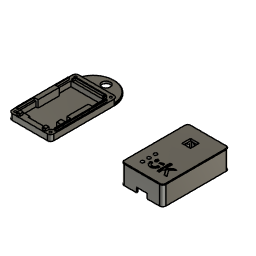
krabka_adam_v7 (Autodesk Fusion 360 design; units mm, degrees)
Autodesk Fusion 360 part; units mm, degrees
sketch "Sketch1" plane through (0, 0, 0) normal (0, 0, 1) x (1, 0, 0)
  line L0 (3.8, 1.2) -> (3.8, 2.7)
  line L1 (3.8, 2.7) -> (10.8, 2.7)
  line L2 (10.8, 2.7) -> (10.8, 1.2)
  line L3 (32.3, 10.7) -> (28, 10.7)
  line L4 (28, 10.7) -> (28, 14.9)
  line L5 (28, 14.9) -> (32.3, 14.9)
  line L6 (1.2, 50.8) -> (32.3, 50.8)
  line L7 (-0.4, 38) -> (3.2, 38)
  line L8 (3.2, 38) -> (3.2, 18)
  line L9 (3.2, 18) -> (-0.4, 18)
  line L10 (33.9, 18) -> (30.3, 18)
  line L11 (30.3, 18) -> (30.3, 38)
  line L12 (30.3, 38) -> (33.9, 38)
  line L13 (1.2, 50.8) -> (1.2, 38)
  line L14 (1.2, 18) -> (1.2, 2.5284)
  line L15 (32.3, 38) -> (32.3, 50.8)
  line L16 (32.3, 14.9) -> (32.3, 18)
  line L17 (2.7981, 1.2) -> (3.8, 1.2)
  line L18 (1.6, 53.5467) -> (1.6, 51.2)
  line L19 (1.6, 51.2) -> (2.8, 51.2)
  line L20 (2.8, 51.2) -> (2.8, 53.2)
  line L21 (2.8, 53.2) -> (30.7, 53.2)
  line L22 (30.7, 53.2) -> (30.7, 51.2)
  line L23 (30.7, 51.2) -> (31.9, 51.2)
  line L24 (31.9, 51.2) -> (31.9, 53.5467)
  line L25 (30.9, 54.4) -> (2.6, 54.4)
  circle A0 centre (33.3, -0.3) radius 2
  circle A1 centre (0.2, -0.3) radius 2
  line L26 (0.2, -3.3) -> (33.3, -3.3)
  circle A2 centre (33.3, 56.2) radius 2
  circle A3 centre (0.2, 56.2) radius 2
  line L27 (0.2, 59.2) -> (33.3, 59.2)
  line L28 (36.3, 56.2) -> (36.3, -0.3)
  line L29 (-2.8, -0.3) -> (-2.8, 56.2)
  arc A4 (32.3, 2.5284) -> (30.7019, 1.2) centre (33.3, -0.3) ccw
  arc A5 (33.3, -3.3) -> (36.3, -0.3) centre (33.3, -0.3) ccw
  line L30 (10.8, 1.2) -> (30.7019, 1.2)
  line L31 (32.3, 2.5284) -> (32.3, 10.7)
  arc A6 (2.7981, 1.2) -> (1.2, 2.5284) centre (0.2, -0.3) ccw
  arc A7 (-2.8, -0.3) -> (0.2, -3.3) centre (0.2, -0.3) ccw
  arc A8 (0.2, 59.2) -> (-2.8, 56.2) centre (0.2, 56.2) ccw
  arc A9 (1.6, 53.5467) -> (2.6, 54.4) centre (0.2, 56.2) ccw
  arc A10 (30.9, 54.4) -> (31.9, 53.5467) centre (33.3, 56.2) ccw
  arc A11 (36.3, 56.2) -> (33.3, 59.2) centre (33.3, 56.2) ccw
  line L32 (3.2, 53.2) -> (30.3, 53.2)
  line L33 (30.3, 1.2) -> (3.2, 1.2)
  circle A12 centre (33.3, 56.2) radius 1.05
  circle A13 centre (0.2, 56.2) radius 1.05
  circle A14 centre (0.2, -0.3) radius 1.05
  circle A15 centre (33.3, -0.3) radius 1.05
  circle A16 centre (16.75, 68.2) radius 4
  line L34 (16.75, 59.2) -> (16.75, 68.2) construction
  arc A17 (36.3, 56.2) -> (-2.8, 56.2) centre (16.75, 56.2) ccw
  line L35 (35.1, 50.8) -> (35.1, 2.5284)
  line L36 (-1.6, 2.5284) -> (-1.6, 50.8)
  line L37 (-0.4, 50.8) -> (-1.6, 50.8)
  line L38 (-0.4, 2.5284) -> (-1.6, 2.5284)
  line L39 (33.9, 50.8) -> (35.1, 50.8)
  line L40 (33.9, 2.5284) -> (35.1, 2.5284)
  line L41 (3.2, -0.9) -> (3.2, -2.1)
  line L42 (30.3, -0.9) -> (30.3, -2.1)
  line L43 (33.9, 50.8) -> (33.9, 38)
  line L44 (33.9, 18) -> (33.9, 2.5284)
  line L45 (-0.4, 2.5284) -> (-0.4, 18)
  line L46 (-0.4, 38) -> (-0.4, 50.8)
  line L47 (3.2, -0.9) -> (3.2, 1.2)
  line L48 (30.3, -0.9) -> (30.3, 1.2)
  line L49 (141.3, 56.2) -> (141.3, -0.3)
  line L50 (102.2, -0.3) -> (102.2, 56.2)
  arc A18 (138.3, -3.3) -> (141.3, -0.3) centre (138.3, -0.3) ccw
  line L51 (105.2, -3.3) -> (138.3, -3.3)
  arc A19 (141.3, 56.2) -> (138.3, 59.2) centre (138.3, 56.2) ccw
  line L52 (105.2, 59.2) -> (138.3, 59.2)
  arc A20 (105.2, 59.2) -> (102.2, 56.2) centre (105.2, 56.2) ccw
  arc A21 (102.2, -0.3) -> (105.2, -3.3) centre (105.2, -0.3) ccw
  circle A22 centre (138.3, -0.3) radius 0.95
  circle A23 centre (105.2, -0.3) radius 0.95
  circle A24 centre (105.2, 56.2) radius 0.95
  circle A25 centre (138.3, 56.2) radius 0.95
  line L53 (103.4, 1.5) -> (103.4, 54.4)
  line L54 (107, -2.1) -> (136.5, -2.1)
  line L55 (140.1, 54.4) -> (140.1, 1.5)
  line L56 (107, 58) -> (136.5, 58)
  line L57 (105.2, 1.5) -> (103.4, 1.5)
  line L58 (107, -0.3) -> (107, -2.1)
  arc A26 (107, -0.3) -> (105.2, 1.5) centre (105.2, -0.3) ccw
  line L59 (140.1, 1.5) -> (138.3, 1.5)
  line L60 (136.5, -0.3) -> (136.5, -2.1)
  arc A27 (138.3, 1.5) -> (136.5, -0.3) centre (138.3, -0.3) ccw
  line L61 (140.1, 54.4) -> (138.3, 54.4)
  line L62 (136.5, 56.2) -> (136.5, 58)
  arc A28 (136.5, 56.2) -> (138.3, 54.4) centre (138.3, 56.2) ccw
  line L63 (107, 58) -> (107, 56.2)
  line L64 (105.2, 54.4) -> (103.4, 54.4)
  arc A29 (105.2, 54.4) -> (107, 56.2) centre (105.2, 56.2) ccw
  circle A30 centre (112.35, 6.7) radius 1.55
  circle A31 centre (112.35, 12.8) radius 1.55
  circle A32 centre (112.35, 18.9) radius 1.55
  line L65 (116, 48) -> (124, 48)
  line L66 (124, 48) -> (124, 40)
  line L67 (124, 40) -> (116, 40)
  line L68 (116, 40) -> (116, 48)
  line L69 (6.2, 1.2) -> (6.2, -2.1)
  line L70 (27.3, 1.2) -> (27.3, -2.1)
  line L71 (3.2, -2.1) -> (6.2, -2.1)
  line L72 (27.3, -2.1) -> (30.3, -2.1)
  dimension "d9" = 2.6
  dimension "d10" = 7
  dimension "d11" = 1.5
  dimension "d12" = 9.5
  dimension "d14" = 4.2
  dimension "d16" = 2
  dimension "d18" = 20
  dimension "d19" = 20
  dimension "d20" = 16.8
  dimension "d21" = 16.8
  dimension "d28" = 1.2
  dimension "d29" = 1.2
  dimension "d32" = 1.2
  dimension "d35" = 2.4
  dimension "d37" = 0.4
  dimension "d46" = 6
  dimension "d47" = 4
  dimension "d48" = 6
  dimension "d49" = 4
  dimension "d50" = 6
  dimension "d51" = 4
  dimension "d52" = 6
  dimension "d53" = 4
  dimension "d54" = 0.3606
  dimension "d55" = 0.2
  dimension "d56" = 2.8
  dimension "d57" = 33.1
  dimension "d58" = 4
  dimension "d59" = 8.3
  dimension "d61" = 4
  dimension "d62" = 56.5
  dimension "d63" = 3
  dimension "d64" = 4.4
  dimension "d66" = 4
  dimension "d67" = 4.4
  dimension "d72" = 2.1
  dimension "d73" = 2.1
  dimension "d74" = 2.1
  dimension "d75" = 2.1
  dimension "d81" = 8
  dimension "d83" = 9
  dimension "d88" = 1.2
  dimension "d89" = 2.8284
  dimension "d90" = 5.4
  dimension "d92" = 1.2
  dimension "d93" = 2.8284
  dimension "d94" = 5.4
  dimension "d95" = 1.2
  dimension "d97" = 3
  dimension "d98" = 3
  dimension "d100" = 3.6
  dimension "d156" = 105.2
  dimension "d157" = 56.2
  dimension "d158" = 105.2
  dimension "d159" = 3
  dimension "d160" = 3
  dimension "d161" = 3
  dimension "d162" = 3
  dimension "d178" = 56.5
  dimension "d179" = 33.1
  dimension "d180" = 56.5
  dimension "d181" = 33.1
  dimension "d182" = 39.1
  dimension "d183" = 62.5
  dimension "d184" = 33.1
  dimension "d185" = 33.1
  dimension "d186" = 1.9
  dimension "d187" = 1.9
  dimension "d188" = 1.9
  dimension "d189" = 1.9
  dimension "d201" = 10.15
  dimension "d202" = 3.1
  dimension "d203" = 10
  dimension "d204" = 6.1
  dimension "d205" = 6.1
  dimension "d206" = 10.15
  dimension "d207" = 10.15
  dimension "d209" = 13.8
  dimension "d210" = 8
  dimension "d211" = 8
  dimension "d214" = 43.3
  dimension "d224" = 3
  dimension "d225" = 3
  constraint perpendicular L0 L17
  constraint perpendicular L0 L1
  constraint coincident L2.end L17
  constraint perpendicular L2 L17
  constraint perpendicular L3 L4
  constraint perpendicular L4 L5
  constraint perpendicular L7 L13
  constraint perpendicular L7 L8
  constraint coincident L14.start L13
  constraint perpendicular L9 L13
  constraint perpendicular L10 L11
  constraint collinear L13 L14
  constraint collinear L17 L30
  constraint perpendicular L6 L18
  constraint perpendicular L18 L19
  constraint perpendicular L19 L20
  constraint perpendicular L20 L21
  constraint perpendicular L21 L22
  constraint perpendicular L22 L23
  constraint perpendicular L23 L24
  constraint horizontal L25
  constraint equal L20 L22
  constraint tangent L11 A4
  constraint tangent L1 A4
  constraint concentric A0 A4
  constraint concentric A1 A6
  constraint tangent L1 A6
  constraint tangent L8 A6
  constraint horizontal L26
  constraint tangent L26 A6
  constraint coincident L26.end A4
  constraint concentric A2 A10
  constraint concentric A3 A8
  constraint tangent L11 A10
  constraint tangent L21 A10
  constraint tangent L21 A8
  constraint tangent L8 A8
  constraint vertical L29
  constraint horizontal L27
  constraint vertical L28
  constraint tangent L28 A4
  constraint tangent L27 A10
  constraint tangent L29 A8
  constraint coincident L29.start A6
  constraint coincident L28.start A10
  constraint concentric A4 A5
  constraint concentric A6 A7
  constraint concentric A8 A9
  constraint concentric A10 A11
  constraint horizontal L32
  constraint horizontal L33
  constraint coincident L30 L33.start
  constraint coincident L21 L32.start
  constraint concentric A11 A12
  constraint concentric A8 A13
  constraint concentric A7 A14
  constraint concentric A4 A15
  constraint midpoint L27 L34.start
  constraint coincident A16.centre L34.end
  constraint perpendicular L27 L34
  constraint tangent A11 A17
  constraint perpendicular L36 L37
  constraint perpendicular L36 L38
  constraint perpendicular L35 L39
  constraint perpendicular L35 L40
  constraint perpendicular L41 L71
  constraint perpendicular L42 L71
  constraint coincident L7.start L45
  constraint coincident L13.end L7
  constraint coincident L14.start L9
  constraint coincident L10.start L43
  constraint coincident L16.end L10
  constraint coincident L15.start L12
  constraint collinear L43 L44
  constraint collinear L45 L46
  constraint perpendicular L33 L47
  constraint perpendicular L30 L48
  constraint horizontal L51
  constraint horizontal L52
  constraint vertical L49
  constraint tangent L50 A20
  constraint concentric A18 A22
  constraint concentric A21 A23
  constraint concentric A20 A24
  constraint concentric A19 A25
  constraint concentric A20 A29
  constraint concentric A21 A26
  constraint concentric A18 A27
  constraint concentric A19 A28
  constraint tangent L55 A27
  constraint tangent L54 A26
  constraint tangent L56 A29
  constraint tangent L53 A29
  constraint tangent L53 A26
  constraint tangent L54 A27
  constraint tangent L55 A28
  constraint tangent L56 A28
  constraint perpendicular L53 L57
  constraint perpendicular L54 L58
  constraint tangent L58 A26
  constraint tangent L57 A26
  constraint perpendicular L55 L59
  constraint perpendicular L54 L60
  constraint tangent L59 A27
  constraint tangent L60 A27
  constraint perpendicular L55 L61
  constraint perpendicular L56 L62
  constraint tangent L62 A28
  constraint tangent L61 A28
  constraint perpendicular L56 L63
  constraint perpendicular L53 L64
  constraint tangent L64 A29
  constraint tangent L63 A29
  constraint equal A30 A31
  constraint equal A30 A32
  constraint horizontal L65
  constraint vertical L66
  constraint horizontal L67
  constraint vertical L68
  constraint coincident L33 L69.start
  constraint perpendicular L69 L71
  constraint coincident L33 L70.start
  constraint coincident L70.end L71
  constraint perpendicular L70 L71
  constraint collinear L71 L72
  measures "d9" distance of L0 L13
  measures "d10" distance of L0.end L1.end
  measures "d11" distance of L1 L17
  measures "d12" distance of L3 L17
  measures "d14" distance of L3.end L4.end
  measures "d16" distance of L8 L13
  measures "d18" distance of L7.end L8.end
  measures "d19" distance of L10.end L11.end
  measures "d20" distance of L9 L17
  measures "d21" distance of L10 L17
  measures "d28" distance of L18 L20
  measures "d29" distance of L22 L24
  measures "d32" distance of L21 L25
  measures "d35" distance of L6 L21
  measures "d37" distance of L6 L23
  measures "d46" diameter of A4
  measures "d47" diameter of A0
  measures "d48" diameter of A6
  measures "d49" diameter of A1
  measures "d50" diameter of A10
  measures "d51" diameter of A2
  measures "d52" diameter of A8
  measures "d53" diameter of A3
  measures "d54" distance of origin A1.centre
  measures "d55" horizontal distance of origin A1.centre
  measures "d56" distance of origin L29
  measures "d57" distance of A1.centre A0.centre
  measures "d58" distance of L28 L31
  measures "d59" distance of L4 L28
  measures "d61" distance of L16 L28
  measures "d62" distance of A0.centre A2.centre
  measures "d63" radius of A9
  measures "d64" distance of L24 L28
  measures "d66" distance of L15 L28
  measures "d67" distance of L18 L29
  measures "d72" diameter of A12
  measures "d73" diameter of A13
  measures "d74" diameter of A14
  measures "d75" diameter of A15
  measures "d81" diameter of A16
  measures "d83" distance of L27 A16.centre
  measures "d88" distance of L36 L45
  measures "d89" distance of A1.centre L38
  measures "d90" distance of A3.centre L37
  measures "d92" distance of L35 L43
  measures "d93" distance of A0.centre L40
  measures "d94" distance of A2.centre L39
  measures "d95" distance of L26 L71
  measures "d97" distance of A1.centre L41
  measures "d98" distance of A0.centre L42
  measures "d100" distance of L11.end L12.end
  measures "d156" horizontal distance of origin A21.centre
  measures "d157" vertical distance of origin A20.centre
  measures "d158" horizontal distance of origin A20.centre
  measures "d159" radius of A20
  measures "d160" radius of A21
  measures "d161" radius of A18
  measures "d162" radius of A19
  measures "d178" distance of A21.centre A20.centre
  measures "d179" distance of A18.centre A21.centre
  measures "d180" distance of A18.centre A19.centre
  measures "d181" distance of A20.centre A19.centre
  measures "d182" distance of L49 L50
  measures "d183" distance of L51 L52
  measures "d184" distance of L51.start A18.start
  measures "d185" distance of L52.start A19.end
  measures "d186" diameter of A22
  measures "d187" diameter of A23
  measures "d188" diameter of A24
  measures "d189" diameter of A25
  measures "d201" distance of L50 A30.centre
  measures "d202" diameter of A30
  measures "d203" distance of L51 A30.centre
  measures "d204" vertical distance of A30.centre A31.centre
  measures "d205" distance of A31.centre A32.centre
  measures "d206" distance of L50 A31.centre
  measures "d207" distance of L50 A32.centre
  measures "d209" distance of L50 L68
  measures "d210" distance of L65 L67
  measures "d211" distance of L66 L68
  measures "d214" distance of L51 L67
  measures "d224" distance of L48 L70
  measures "d225" distance of L47 L69
extrude "Extrude6" add sketch "Sketch1" along normal blind 6 contours L17 L33 L41 L47 L69 L71 | L0 L1 L2 L33 | L30 L33 L42 L48 L70 L72 | L7 L8 L9 L36 L37 L38 L45 L46 | L10 L11 L12 L35 L39 L40 L43 L44 | L18 L19 L20 L21 L22 L23 L24 L25 A9 A10 L32 | L26 L27 L28 L29 A5 A7 A8 A11 makes body 1
extrude "Extrude7" add sketch "Sketch1" along normal blind 8 contours L17 L33 L41 L47 L69 L71 | L30 L33 L42 L48 L70 L72 | L7 L8 L9 L36 L37 L38 L45 L46 | L10 L11 L12 L35 L39 L40 L43 L44 | L18 L19 L20 L21 L22 L23 L24 L25 A9 A10 L32 bodies 1
extrude "Extrude8" add sketch "Sketch1" along normal blind 3.8 from surface at 2.2 contours A0 | A1 | A2 | A3 bodies 1
extrude "Extrude9" add sketch "Sketch1" along normal blind 1.2 contours L0 L1 L2 L3 L4 L5 L6 L7 L8 L9 L10 L11 L12 L13 L14 L15 L16 L17 A4 L30 L31 A6 L33 bodies 1
extrude "Extrude10" add sketch "Sketch1" along normal blind 2 contours L27 A8 A11 A17 bodies 1
chamfer "Chamfer1" distance 0.5 angle 45 6 edges at (36.3, 27.95, 0) (35.4213, -2.4213, 0) (16.75, -3.3, 0) (-1.9213, -2.4213, 0) (-2.8, 27.95, 0) (16.75, 75.75, 0) on bodies 1
chamfer "Chamfer1" distance 0.5 angle 45 1 edges at (16.75, 75.75, 2) on bodies 1
chamfer "Chamfer2" distance 0.5 angle 45 9 edges at (35.1, 26.6642, 8) (4.7, -2.1, 8) (28.8, -2.1, 8) (-1.6, 26.6642, 8) (16.75, 54.4, 8) (31.9, 52.3734, 8) (31.3527, 53.9179, 8) (2.1473, 53.9179, 8) (1.6, 52.3734, 8) on bodies 1
extrude "Extrude11" add sketch "Sketch1" along normal blind 2 from surface at 16 separate body contours L53 L54 L55 L56 L57 L58 A26 L59 L60 A27 L61 L62 A28 L63 L64 A29 makes body 2
extrude "Extrude12" add sketch "Sketch1" along normal blind 18 contours L49 L50 A18 L51 A19 L52 A20 A21 bodies 2
extrude "Extrude13" add sketch "Sketch1" along normal blind 3 from surface at 15 contours A22 | A23 | A24 | A25 bodies 2
sketch "Sketch3" plane through (0, 0, 18) normal (0, 0, 1) x (-1, 0, 0)
  arc A0 (-105.2, -59.2) -> (-102.2, -56.2) centre (-105.2, -56.2) ccw
  line L0 (-102.2, -56.2) -> (-102.2, 0.3)
  arc A1 (-102.2, 0.3) -> (-105.2, 3.3) centre (-105.2, 0.3) ccw
  line L1 (-105.2, 3.3) -> (-138.3, 3.3)
  arc A2 (-138.3, 3.3) -> (-141.3, 0.3) centre (-138.3, 0.3) ccw
  line L2 (-141.3, 0.3) -> (-141.3, -56.2)
  arc A3 (-141.3, -56.2) -> (-138.3, -59.2) centre (-138.3, -56.2) ccw
  line L3 (-138.3, -59.2) -> (-105.2, -59.2)
  line L4 (-124, -40) -> (-116, -40)
  line L5 (-116, -40) -> (-116, -48)
  line L6 (-116, -48) -> (-124, -48)
  line L7 (-124, -48) -> (-124, -40)
  circle A4 centre (-112.35, -18.9) radius 1.55
  circle A5 centre (-112.35, -12.8) radius 1.55
  circle A6 centre (-112.35, -6.7) radius 1.55
  line L8 (-115.8427, -12.1922) -> (-115.8427, -18.4226)
  line L9 (-115.8427, -18.4226) -> (-121.233, -18.4226)
  line L10 (-121.233, -18.4226) -> (-126.6233, -18.4226)
  line L11 (-126.6233, -18.4226) -> (-126.6233, -12.2972)
  line L12 (-126.6233, -12.2972) -> (-126.6233, -6.1718)
  line L13 (-126.6233, -6.1718) -> (-127.6384, -6.1718)
  line L14 (-127.6384, -6.1718) -> (-128.6535, -6.1718)
  line L15 (-128.6535, -6.1718) -> (-128.6535, -7.7829)
  line L16 (-128.6535, -7.7829) -> (-128.6535, -9.394)
  line L17 (-128.6535, -9.394) -> (-129.2896, -10.0055)
  spline S0 degree 3 poles (-129.2896, -10.0055) (-129.6394, -10.3419) (-129.9466, -10.6238) (-129.9721, -10.6319) knots 0 0 0 0 1 1 1 1
  spline S1 degree 3 poles (-129.9721, -10.6319) (-129.9976, -10.6401) (-130.2421, -10.3408) (-130.5154, -9.9669) knots 0 0 0 0 1 1 1 1
  spline S2 degree 3 poles (-130.5154, -9.9669) (-130.7887, -9.593) (-131.5271, -8.5861) (-132.1565, -7.7294) knots 0 0 0 0 1 1 1 1
  line L18 (-132.1565, -7.7294) -> (-133.3007, -6.1718)
  line L19 (-133.3007, -6.1718) -> (-134.5123, -6.1718)
  spline S3 degree 3 poles (-134.5123, -6.1718) (-135.5426, -6.1718) (-135.7239, -6.1561) (-135.7239, -6.0668) knots 0 0 0 0 1 1 1 1
  spline S4 degree 3 poles (-135.7239, -6.0668) (-135.7239, -5.974) (-134.5727, -5.9618) (-125.7833, -5.9618) knots 0 0 0 0 1 1 1 1
  line L20 (-125.7833, -5.9618) -> (-115.8427, -5.9618)
  line L21 (-115.8427, -5.9618) -> (-115.8427, -12.1922)
  spline S5 degree 3 poles (-121.399, -6.1362) (-122.2006, -6.306) (-122.8682, -6.6822) (-123.5081, -7.3247) knots 0 0 0 0 1 1 1 1
  spline S6 degree 3 poles (-123.5081, -7.3247) (-124.3306, -8.1504) (-124.6782, -8.9335) (-124.7599, -10.1446) knots 0 0 0 0 1 1 1 1
  line L22 (-124.7599, -10.1446) -> (-124.7988, -10.7221)
  line L23 (-124.7988, -10.7221) -> (-123.7605, -10.7221)
  line L24 (-123.7605, -10.7221) -> (-122.7222, -10.7221)
  line L25 (-122.7222, -10.7221) -> (-122.6875, -10.0602)
  spline S7 degree 3 poles (-122.6875, -10.0602) (-122.6321, -9.0009) (-122.2578, -8.4125) (-121.3762, -7.999) knots 0 0 0 0 1 1 1 1
  spline S8 degree 3 poles (-121.3762, -7.999) (-121.0433, -7.8429) (-120.8931, -7.8169) (-120.3219, -7.8169) knots 0 0 0 0 1 1 1 1
  spline S9 degree 3 poles (-120.3219, -7.8169) (-119.7105, -7.8169) (-119.6174, -7.8358) (-119.1883, -8.0469) knots 0 0 0 0 1 1 1 1
  spline S10 degree 3 poles (-119.1883, -8.0469) (-118.3974, -8.4359) (-118.0175, -9.0706) (-117.9588, -10.1013) knots 0 0 0 0 1 1 1 1
  line L26 (-117.9588, -10.1013) -> (-117.924, -10.7119)
  line L27 (-117.924, -10.7119) -> (-117.4258, -10.7571)
  spline S11 degree 3 poles (-117.4258, -10.7571) (-117.1519, -10.7819) (-116.7072, -10.7921) (-116.4377, -10.7797) knots 0 0 0 0 1 1 1 1
  line L28 (-116.4377, -10.7797) -> (-115.9477, -10.7571)
  line L29 (-115.9477, -10.7571) -> (-115.9527, -10.1217)
  spline S12 degree 3 poles (-115.9527, -10.1217) (-115.9619, -8.9519) (-116.2911, -8.171) (-117.136, -7.3146) knots 0 0 0 0 1 1 1 1
  spline S13 degree 3 poles (-117.136, -7.3146) (-117.7707, -6.6712) (-118.3969, -6.3164) (-119.2079, -6.1405) knots 0 0 0 0 1 1 1 1
  spline S14 degree 3 poles (-119.2079, -6.1405) (-119.8026, -6.0116) (-120.8016, -6.0096) (-121.399, -6.1361) knots 0 0 0 0 1 1 1 1
  line L30 (-121.399, -6.1361) -> (-121.399, -6.1362)
  spline S15 degree 3 poles (-118.4353, -12.7518) (-118.7578, -12.8414) (-119.1688, -13.2675) (-119.3049, -13.6536) knots 0 0 0 0 1 1 1 1
  spline S16 degree 3 poles (-119.3049, -13.6536) (-119.5496, -14.3477) (-119.3519, -15.2268) (-118.8575, -15.6428) knots 0 0 0 0 1 1 1 1
  spline S17 degree 3 poles (-118.8575, -15.6428) (-117.7656, -16.5616) (-116.4588, -14.9288) (-117.1377, -13.4939) knots 0 0 0 0 1 1 1 1
  spline S18 degree 3 poles (-117.1377, -13.4939) (-117.3442, -13.0573) (-117.4897, -12.9124) (-117.8507, -12.7837) knots 0 0 0 0 1 1 1 1
  spline S19 degree 3 poles (-117.8507, -12.7837) (-118.1784, -12.6668) (-118.1374, -12.669) (-118.4353, -12.7518) knots 0 0 0 0 1 1 1 1
  spline S20 degree 3 poles (-122.7519, -13.2792) (-124.29, -13.4482) (-124.8198, -13.5156) (-124.8501, -13.5459) knots 0 0 0 0 1 1 1 1
  spline S21 degree 3 poles (-124.8501, -13.5459) (-124.8734, -13.5691) (-124.5803, -14.8903) (-124.4874, -15.1807) knots 0 0 0 0 1 1 1 1
  spline S22 degree 3 poles (-124.4874, -15.1807) (-124.4694, -15.2371) (-123.9446, -15.0924) (-122.8644, -14.7335) knots 0 0 0 0 1 1 1 1
  spline S23 degree 3 poles (-122.8644, -14.7335) (-121.9864, -14.4417) (-121.2547, -14.1914) (-121.2385, -14.1773) knots 0 0 0 0 1 1 1 1
  spline S24 degree 3 poles (-121.2385, -14.1773) (-121.2037, -14.1471) (-121.3637, -13.244) (-121.4199, -13.1531) knots 0 0 0 0 1 1 1 1
  spline S25 degree 3 poles (-121.4199, -13.1531) (-121.441, -13.1189) (-121.5319, -13.1094) (-121.6219, -13.132) knots 0 0 0 0 1 1 1 1
  spline S26 degree 3 poles (-121.6219, -13.132) (-121.7119, -13.1546) (-122.2204, -13.2208) (-122.7519, -13.2792) knots 0 0 0 0 1 1 1 1
  spline S27 degree 3 poles (-134.5821, -7.8023) (-133.9734, -8.6574) (-133.3848, -9.483) (-133.2742, -9.637) knots 0 0 0 0 1 1 1 1
  spline S28 degree 3 poles (-133.2742, -9.637) (-133.1635, -9.7911) (-132.7231, -10.4053) (-132.2955, -11.0021) knots 0 0 0 0 1 1 1 1
  line L31 (-132.2955, -11.0021) -> (-131.5181, -12.0872)
  line L32 (-131.5181, -12.0872) -> (-132.1783, -12.7172)
  spline S29 degree 3 poles (-132.1783, -12.7172) (-132.5415, -13.0638) (-133.4091, -13.8795) (-134.1063, -14.53) knots 0 0 0 0 1 1 1 1
  spline S30 degree 3 poles (-134.1063, -14.53) (-134.8034, -15.1805) (-135.3739, -15.7239) (-135.3739, -15.7376) knots 0 0 0 0 1 1 1 1
  spline S31 degree 3 poles (-135.3739, -15.7376) (-135.3739, -15.7512) (-134.7966, -15.7624) (-134.0911, -15.7624) knots 0 0 0 0 1 1 1 1
  line L33 (-134.0911, -15.7624) -> (-132.8084, -15.7624)
  line L34 (-132.8084, -15.7624) -> (-132.3627, -15.3599)
  spline S32 degree 3 poles (-132.3627, -15.3599) (-132.1175, -15.1385) (-131.4721, -14.5478) (-130.9283, -14.0473) knots 0 0 0 0 1 1 1 1
  spline S33 degree 3 poles (-130.9283, -14.0473) (-130.3846, -13.5468) (-129.6503, -12.8751) (-129.2966, -12.5547) knots 0 0 0 0 1 1 1 1
  line L35 (-129.2966, -12.5547) -> (-128.6535, -11.9721)
  line L36 (-128.6535, -11.9721) -> (-128.6535, -15.1973)
  line L37 (-128.6535, -15.1973) -> (-128.6535, -18.4226)
  line L38 (-128.6535, -18.4226) -> (-132.1887, -18.4226)
  line L39 (-132.1887, -18.4226) -> (-135.7239, -18.4226)
  line L40 (-135.7239, -18.4226) -> (-135.7239, -12.3322)
  spline S34 degree 3 poles (-135.7239, -12.3322) (-135.7239, -8.9825) (-135.716, -6.2431) (-135.7064, -6.2447) knots 0 0 0 0 1 1 1 1
  spline S35 degree 3 poles (-135.7064, -6.2447) (-135.6968, -6.2463) (-135.1909, -6.9472) (-134.5821, -7.8023) knots 0 0 0 0 1 1 1 1
  line L41 (-115.8427, -18.4226) -> (-135.7239, -18.4226)
  line L42 (-135.7239, -18.4226) -> (-135.7239, -6.0668)
  line L43 (-135.7239, -6.0668) -> (-115.8427, -6.0668)
  line L44 (-115.8427, -6.0668) -> (-115.8427, -18.4226)
  line L45 (-135.5866, -6.1435) -> (-135.7113, -6.4868)
  constraint horizontal L41
  constraint vertical L42
  constraint horizontal L43
  constraint vertical L44
  constraint coincident S3 L45.start
  constraint coincident S34 L45.end
extrude "Extrude14" cut sketch "Sketch3" against normal blind 1 contours S5 S6 L22 L23 L24 L25 S7 S8 S9 S10 L26 L27 S11 L28 L29 S12 S13 S14 L43 | L11 L12 L13 L14 L15 L16 L17 S0 S1 S2 L18 L19 S3 S27 S28 L31 L32 S29 S30 S31 L33 L34 S32 S33 L35 L36 L37 S35 L41 L45 | S15 S16 S17 S18 S19 | S20 S21 S22 S23 S24 S25 S26 bodies 2
sketch "Sketch4" plane through (0, -3.3, 0) normal (0, -1, 0) x (1, 0, 0)
  line L0 (105.2, 0) -> (138.3, 0)
  line L1 (138.3, 0) -> (138.3, 18)
  line L2 (138.3, 18) -> (105.2, 18)
  line L3 (105.2, 18) -> (105.2, 0)
  line L4 (121.75, 0) -> (121.75, 4.5) construction
  line L5 (116.85, 4.5) -> (126.65, 4.5)
  line L6 (116.85, 4.5) -> (116.85, 0)
  line L7 (126.65, 4.5) -> (126.65, 0)
  dimension "d215" = 4.5
  dimension "d216" = 9.8
  constraint midpoint L0 L4.start
  constraint perpendicular L0 L4
  constraint perpendicular L3 L5
  constraint midpoint L4.end L5
  constraint coincident L0 L6.end
  constraint perpendicular L0 L6
  constraint coincident L0 L7.end
  constraint perpendicular L0 L7
  measures "d215" distance of L4.start L4.end
  measures "d216" distance of L5.start L5.end
extrude "Extrude15" cut sketch "Sketch4" against normal blind 1.2 contours L0 L5 L6 L7 bodies 2
sketch "Sketch5" plane through (0, 59.2, 0) normal (0, 1, 0) x (-1, 0, 0)
  line L0 (-138.3, 0) -> (-105.2, 0)
  line L1 (-105.2, 0) -> (-105.2, 18)
  line L2 (-105.2, 18) -> (-138.3, 18)
  line L3 (-138.3, 18) -> (-138.3, 0)
  circle A0 centre (-111.7, 7.5) radius 3.5
  line L4 (-102.2, 0) -> (-102.2, 18)
  dimension "d219" = 9.5
  dimension "d220" = 7
  dimension "d221" = 7.5
  measures "d219" distance of A0.centre L4
  measures "d220" diameter of A0
  measures "d221" distance of L0 A0.centre
extrude "Extrude16" cut sketch "Sketch5" against normal blind 1.2 contours A0 bodies 2
sketch "Sketch6" plane through (0, 0, 16) normal (0, 0, -1) x (1, 0, 0)
  circle A0 centre (112.35, -18.9) radius 1.55
  line L0 (116, -40) -> (124, -40)
  line L1 (124, -40) -> (124, -48)
  line L2 (124, -48) -> (116, -48)
  line L3 (116, -48) -> (116, -40)
  circle A1 centre (112.35, -12.8) radius 1.55
  circle A2 centre (112.35, -6.7) radius 1.55
  line L4 (107, 2.1) -> (107, 0.3)
  arc A3 (105.2, -1.5) -> (107, 0.3) centre (105.2, 0.3) ccw
  line L5 (105.2, -1.5) -> (103.4, -1.5)
  line L6 (103.4, -1.5) -> (103.4, -54.4)
  line L7 (103.4, -54.4) -> (105.2, -54.4)
  arc A4 (107, -56.2) -> (105.2, -54.4) centre (105.2, -56.2) ccw
  line L8 (107, -56.2) -> (107, -58)
  line L9 (107, -58) -> (136.5, -58)
  line L10 (136.5, -58) -> (136.5, -56.2)
  arc A5 (138.3, -54.4) -> (136.5, -56.2) centre (138.3, -56.2) ccw
  line L11 (138.3, -54.4) -> (140.1, -54.4)
  line L12 (140.1, -54.4) -> (140.1, -1.5)
  line L13 (140.1, -1.5) -> (138.3, -1.5)
  arc A6 (136.5, 0.3) -> (138.3, -1.5) centre (138.3, 0.3) ccw
  line L14 (136.5, 0.3) -> (136.5, 2.1)
  line L15 (136.5, 2.1) -> (107, 2.1)
  circle A7 centre (112, -50) radius 1
  circle A8 centre (128, -50) radius 1
  line L16 (112, -50) -> (128, -50) construction
  line L17 (120, -48) -> (120, -50) construction
  dimension "d226" = 2
  dimension "d227" = 16
  dimension "d228" = 8
  constraint equal A7 A8
  constraint coincident A7.centre L16.start
  constraint coincident A8.centre L16.end
  constraint horizontal L16
  constraint midpoint L2 L17.start
  constraint midpoint L16 L17.end
  constraint perpendicular L16 L17
  measures "d226" diameter of A8
  measures "d227" distance of A7.centre A8.centre
  measures "d228" distance of L9 A8.centre
extrude "Extrude17" add sketch "Sketch6" along normal blind 5 contours A7 | A8 bodies 2
chamfer "Chamfer3" distance 0.5 angle 45 8 edges at (141.3, 27.95, 18) (140.4213, 58.3213, 18) (121.75, 59.2, 18) (103.0787, 58.3213, 18) (102.2, 27.95, 18) (103.0787, -2.4213, 18) (121.75, -3.3, 18) (140.4213, -2.4213, 18) on bodies 2
equation "d198 = 22 mm - 7 mm"
equation "d201 = ( 5.6 / 2 ) * 1 mm + 5.8 mm + ( 3.1 / 2 ) * 1 mm"
equation "d204 = 3 mm + 3.1 mm"
equation "d205 = d204"
equation "d206 = d201"
equation "d207 = d206"
equation "d209 = ( 5.6 / 2 ) * 1 mm + 11 mm"
equation "d214 = 40 mm + 4.5 mm - 1.2 mm"
equation "d219 = 2.8 mm + 2.2 mm + mm + d220 / 2"
equation "d221 = 4 mm + d220 / 2"
